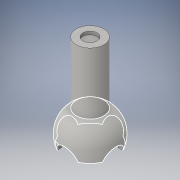
# Autodesk Inventor part: caster sumo jeffrey p
Saved by Autodesk Inventor 2016 (Build 200138000, 138)
## iProperties
Created: 2017-09-07
Part Number: caster sumo jeffrey p
Material: Generic
Document SubType Name: Modeling
Designer: student
Density: 1 g/cm^3
Appearance: Default
Author: student
Autodesk Inventor part; units mm, degrees
ref_plane "YZ Plane" through (0, 0, 0) normal (1, 0, 0) x (0, 1, 0)
ref_plane "XZ Plane" through (0, 0, 0) normal (0, 1, 0) x (-1, 0, 0)
ref_plane "XY Plane" through (0, 0, 0) normal (0, 0, 1) x (1, 0, 0)
sketch "Sketch1" plane through (0, 0, 0) normal (0, 0, 1) x (1, 0, 0)
  arc A0 (-5.5597, 8.9556) -> (-9.9691, -3.4248) centre (0, 0) ccw
  line L0 (0, 0) -> (0, 33.782)
  line L1 (0, 33.782) -> (-5.5597, 33.782)
  line L2 (-5.5597, 33.782) -> (-5.5597, 8.9556)
  line L3 (0, 0) -> (0, -2.735)
  arc A1 (0, 9.017) -> (-8.3413, -3.4248) centre (0, 0) ccw
  line L4 (-9.9691, -3.4248) -> (-8.3413, -3.4248)
  dimension "d1" = 21.082
  dimension "d2" = 1.524
  dimension "d12" = 33.782
  constraints: 10 end point, 4 point on circle, 2 centre point, 2 coincident, 2 perpendicular, 2 vertical, 1 horizontal, 1 point on line
  measures "d1" diameter of A0
  measures "d2" radial gap between concentric circles of A1 A0
  measures "d12" distance of L0.start L0.end
revolve "Revolution1" add sketch "Sketch1" angle 360 about axis through (0, 0, 0) along (0, 1, 0)
sketch "Sketch4" plane through (0, 33.782, 0) normal (0, 1, 0) x (1, 0, 0)
  circle A0 centre (0, 0) radius 2.8575
  dimension "d4" = 5.715
  constraints: 1 centre point, 1 coincident
  measures "d4" diameter of A0
extrude "Extrusion1" cut sketch "Sketch4" against normal blind 1.27
sketch "Sketch5" plane through (0, 0, 0) normal (1, 0, 0) x (0, 1, 0)
  line L0 (-3.4248, -9.9691) -> (-3.4248, 9.9691) projected
  circle A0 centre (-3.4248, 0) radius 4.064
  point P0 (0, 0)
  dimension "d7" = 8.128
  constraints: 1 centre point, 1 midpoint
  measures "d7" diameter of A0
extrude "Extrusion2" cut sketch "Sketch5" along normal mid plane 2540
sketch "Sketch7" plane through (0, 0, 0) normal (0, 0, 1) x (1, 0, 0)
  line L0 (7.2843, -3.4248) -> (-7.2843, -3.4248) projected
  circle A0 centre (0, -3.4248) radius 4.1452
  point P0 (0, 0)
  constraints: 1 centre point, 1 midpoint
extrude "Extrusion3" cut sketch "Sketch7" along normal mid plane 2540
body "Solid1"
